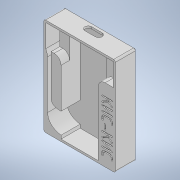
# Autodesk Inventor part: Корпус
Saved by Autodesk Inventor 2021.2 (Build 252289000, 289)
## iProperties
Created: 2023-10-18
Part Number: Корпус
Material: Типовые
Document SubType Name: Modeling
Designer: DELL
Density: 1 g/cm^3
Appearance: По умолчанию
Author: DELL
Autodesk Inventor part; units mm, degrees
ref_plane "YZ Plane" through (0, 0, 0) normal (1, 0, 0) x (0, 1, 0)
ref_plane "XZ Plane" through (0, 0, 0) normal (0, 1, 0) x (-1, 0, 0)
ref_plane "XY Plane" through (0, 0, 0) normal (0, 0, 1) x (1, 0, 0)
sketch "Эскиз1" plane through (0, 0, 0) normal (0, 0, 1) x (1, 0, 0)
  line L0 (10.25, -26.5) -> (-10.25, -26.5) construction
  line L1 (-10.25, -26.5) -> (-10.25, 26.5) construction
  line L2 (-10.25, 26.5) -> (10.25, 26.5) construction
  line L3 (10.25, 26.5) -> (10.25, -26.5) construction
  line L4 (10.25, -26.5) -> (-10.25, 26.5) construction
  line L5 (-10.25, -26.5) -> (10.25, 26.5) construction
  line L6 (19, 14.5) -> (-19, 14.5) construction
  line L7 (-19, 14.5) -> (-19, 26.5) construction
  line L8 (-19, 26.5) -> (19, 26.5) construction
  line L9 (19, 26.5) -> (19, 14.5) construction
  line L10 (19, 14.5) -> (-19, 26.5) construction
  line L11 (-19, 14.5) -> (19, 26.5) construction
  line L12 (-19.5, 14) -> (-14.75, 14)
  arc A0 (-10.75, 10) -> (-14.75, 14) centre (-14.75, 10) ccw
  line L13 (-10.75, 10) -> (-10.75, -27)
  line L14 (-10.75, -27) -> (10.75, -27)
  line L15 (10.75, -27) -> (10.75, 10)
  arc A1 (14.75, 14) -> (10.75, 10) centre (14.75, 10) ccw
  line L16 (14.75, 14) -> (19.5, 14)
  line L17 (19.5, 14) -> (19.5, 27)
  line L18 (19.5, 27) -> (-19.5, 27)
  line L19 (-19.5, 27) -> (-19.5, 14)
  line L20 (0, 26.5) -> (0, -26.5) construction
  line L21 (20.7, -28.2) -> (-20.7, -28.2)
  line L22 (-20.7, -28.2) -> (-20.7, 28.2)
  line L23 (-20.7, 28.2) -> (20.7, 28.2)
  line L24 (20.7, 28.2) -> (20.7, -28.2)
  line L25 (20.7, -28.2) -> (-20.7, 28.2) construction
  line L26 (-20.7, -28.2) -> (20.7, 28.2) construction
  line L27 (-10.75, 10) -> (-10.75, 27)
  line L28 (10.75, 10) -> (10.75, 27)
  point P0 (0, 0)
  point P1 (0, 20.5)
  point P2 (0, 20.5)
  point P3 (0, 0)
  point P4 (0, 0)
  dimension "d0" = 20.5
  dimension "d1" = 53
  dimension "d2" = 38
  dimension "d3" = 12
  dimension "d4" = 0
  dimension "d5" = 0.5
  dimension "d8" = 0.5
  dimension "d9" = 0.5
  dimension "d10" = 0.5
  dimension "d11" = 0.5
  dimension "d12" = 4
  dimension "d13" = 1.2
  dimension "d14" = 1.2
  dimension "d15" = 1.2
  constraints: 58 end point, 11 midpoint, 10 perpendicular, 7 parallel, 5 horizontal, 4 point on circle, 4 tangent, 3 point on line, 2 centre point, 1 vertical alignment, 3 other
  measures "d0" distance of L1.end L2.end
  measures "d1" distance of L0.end L1.end
  measures "d2" distance of L7.end L8.end
  measures "d3" distance of L6.end L7.end
  measures "d4" distance between parallel lines of L2 L8
  measures "d5" distance between parallel lines of L19 L7
  measures "d8" distance between parallel lines of L18 L8
  measures "d9" distance between parallel lines of L6 L12
  measures "d10" distance between parallel lines of L1 L13
  measures "d11" distance between parallel lines of L0 L14
  measures "d12" radius of A0
  measures "d13" distance between parallel lines of L23 L18
  measures "d14" distance between parallel lines of L22 L19
  measures "d15" distance between parallel lines of L14 L21
extrude "Выдавливание1" add sketch "Эскиз1" along normal blind 6 contours L19 L18 L27 A0 L12 | L18 L17 L16 A1 L28 | L21 L22 L23 L24
extrude "Выдавливание2" add sketch "Эскиз1" along normal blind 5 from surface at 6
extrude "Выдавливание3" add sketch "Эскиз1" against normal blind 1 contours L19 L18 L27 A0 L12 | L27 L18 L28 L15 L14 L13 | L18 L17 L16 A1 L28 | L21 L22 L23 L24
fillet "Сопряжение1" radius 1 4 edges at (-20.7, 28.2, 5) (20.7, 28.2, 5) (-20.7, -28.2, 5) (20.7, -28.2, 5)
chamfer "Фаска1" distance 0.5 angle 45 8 edges at (20.7, 0, -1) (20.4071, -27.9071, -1) (0, -28.2, -1) (-20.4071, -27.9071, -1) (-20.7, 0, -1) (-20.4071, 27.9071, -1) (0, 28.2, -1) (20.4071, 27.9071, -1)
sketch "Эскиз2" plane through (-19.7, 28.2, 11) normal (0, 1, 0) x (1, 0, 0)
  line L0 (8.95, 11) -> (30.45, 11) construction
  line L1 (8.95, 11) -> (8.95, 5) construction
  line L2 (30.45, 11) -> (30.45, 5) construction
  line L3 (22.7, 8) -> (16.7, 8) construction
  line L4 (22.7, 10) -> (16.7, 10)
  line L5 (16.7, 6) -> (22.7, 6)
  arc A0 (22.7, 6) -> (22.7, 10) centre (22.7, 8) ccw
  arc A1 (16.7, 10) -> (16.7, 6) centre (16.7, 8) ccw
  point P0 (19.7, 11)
  point P1 (19.7, 8)
  point P2 (19.7, 11)
  dimension "d26" = 10
  dimension "d27" = 4
  dimension "d28" = 1
  constraints: 8 end point, 4 point on circle, 4 tangent, 2 centre point, 2 midpoint, 2 parallel, 1 vertical alignment
  measures "d27" distance between parallel lines of L5 L4
  measures "d28" distance between parallel lines of L4 L0
extrude "Выдавливание4" cut sketch "Эскиз2" against normal up to next
sketch "Эскиз3" plane through (-19.7, 28.2, 11) normal (0, 0, 1) x (1, 0, 0)
  line L0 (38.6265, -20.4965) -> (38.6265, -53.3812) construction
  line L1 (38.6265, -53.3812) -> (33.4814, -53.3812) construction
  line L2 (33.4814, -53.3812) -> (33.4814, -20.4965) construction
  line L3 (33.4814, -20.4965) -> (38.6265, -20.4965) construction
  line L4 (39.4, -56.4) -> (0, -56.4) construction
  line L5 (19.7, -56.4) -> (19.7, 0) construction
  line L6 (16.7, 0) -> (22.7, 0) construction
  line L7 (35.6294, -22.5215) -> (34.8335, -21.8566)
  line L8 (34.8335, -21.8566) -> (32.9093, -21.8566)
  spline S0 degree 2 poles (32.9093, -21.8566) (32.5265, -21.8566) (32.5265, -21.4737) knots 0 0 0 1 1 1
  spline S1 degree 2 poles (32.5265, -21.4737) (32.5265, -21.0909) (32.9093, -21.0909) knots 0 0 0 1 1 1
  line L9 (32.9093, -21.0909) -> (38.2487, -21.0909)
  spline S2 degree 2 poles (38.2487, -21.0909) (38.6265, -21.0909) (38.6265, -21.4737) knots 0 0 0 1 1 1
  spline S3 degree 2 poles (38.6265, -21.4737) (38.6265, -21.8566) (38.2487, -21.8566) knots 0 0 0 1 1 1
  line L10 (38.2487, -21.8566) -> (35.841, -21.8566)
  line L11 (35.841, -21.8566) -> (38.5006, -24.1535)
  spline S4 degree 2 poles (38.5006, -24.1535) (38.6265, -24.2643) (38.6265, -24.4406) knots 0 0 0 1 1 1
  spline S5 degree 2 poles (38.6265, -24.4406) (38.6265, -24.8235) (38.2487, -24.8235) knots 0 0 0 1 1 1
  spline S6 degree 2 poles (38.2487, -24.8235) (38.1027, -24.8235) (37.9616, -24.5968) knots 0 0 0 1 1 1
  line L12 (37.9616, -24.5968) -> (36.1684, -23.0453)
  line L13 (36.1684, -23.0453) -> (33.0957, -24.768)
  spline S7 degree 2 poles (33.0957, -24.768) (33.0051, -24.8235) (32.9093, -24.8235) knots 0 0 0 1 1 1
  spline S8 degree 2 poles (32.9093, -24.8235) (32.7582, -24.8235) (32.5265, -24.5867) (32.5265, -24.4406) knots 0 0 0 1 2 2 2
  spline S9 degree 2 poles (32.5265, -24.4406) (32.5265, -24.2089) (32.7733, -24.088) knots 0 0 0 1 1 1
  line L14 (32.7733, -24.088) -> (35.6294, -22.5215)
  spline S10 degree 2 poles (38.6265, -29.1856) (38.6265, -29.5685) (38.2487, -29.5685) knots 0 0 0 1 1 1
  line L15 (38.2487, -29.5685) -> (32.9093, -29.5685)
  spline S11 degree 2 poles (32.9093, -29.5685) (32.5265, -29.5685) (32.5265, -29.1856) knots 0 0 0 1 1 1
  spline S12 degree 2 poles (32.5265, -29.1856) (32.5265, -28.8028) (32.9093, -28.8028) knots 0 0 0 1 1 1
  line L16 (32.9093, -28.8028) -> (36.7779, -28.8028)
  line L17 (36.7779, -28.8028) -> (33.1814, -26.6066)
  spline S13 degree 2 poles (33.1814, -26.6066) (32.8791, -26.6066) (32.7784, -26.5764) knots 0 0 0 1 1 1
  spline S14 degree 2 poles (32.7784, -26.5764) (32.5265, -26.5109) (32.5265, -26.2238) knots 0 0 0 1 1 1
  spline S15 degree 2 poles (32.5265, -26.2238) (32.5265, -25.841) (32.9093, -25.841) knots 0 0 0 1 1 1
  line L18 (32.9093, -25.841) -> (38.2487, -25.841)
  spline S16 degree 2 poles (38.2487, -25.841) (38.6265, -25.841) (38.6265, -26.2238) knots 0 0 0 1 1 1
  spline S17 degree 2 poles (38.6265, -26.2238) (38.6265, -26.6066) (38.2487, -26.6066) knots 0 0 0 1 1 1
  line L19 (38.2487, -26.6066) -> (34.3802, -26.6066)
  line L20 (34.3802, -26.6066) -> (37.9767, -28.8028)
  spline S18 degree 2 poles (37.9767, -28.8028) (38.279, -28.8028) (38.3747, -28.828) knots 0 0 0 1 1 1
  spline S19 degree 2 poles (38.3747, -28.828) (38.6265, -28.8935) (38.6265, -29.1856) knots 0 0 0 1 1 1
  spline S20 degree 2 poles (38.6265, -33.3463) (38.6265, -33.7292) (38.2487, -33.7292) knots 0 0 0 1 1 1
  spline S21 degree 2 poles (38.2487, -33.7292) (37.8659, -33.7292) (37.8659, -33.3463) knots 0 0 0 1 1 1
  line L21 (37.8659, -33.3463) -> (37.8659, -32.1626)
  spline S22 degree 2 poles (37.8659, -32.1626) (37.8659, -31.6992) (37.468, -31.4675) knots 0 0 0 1 1 1
  spline S23 degree 2 poles (37.468, -31.4675) (37.2816, -31.3566) (37.06, -31.3566) knots 0 0 0 1 1 1
  line L22 (37.06, -31.3566) -> (34.0981, -31.3566)
  spline S24 degree 2 poles (34.0981, -31.3566) (33.7606, -31.3566) (33.2871, -31.8301) (33.2871, -32.1626) knots 0 0 0 1 2 2 2
  line L23 (33.2871, -32.1626) -> (33.2871, -33.3463)
  spline S25 degree 2 poles (33.2871, -33.3463) (33.2871, -33.7292) (32.9093, -33.7292) knots 0 0 0 1 1 1
  spline S26 degree 2 poles (32.9093, -33.7292) (32.5265, -33.7292) (32.5265, -33.3463) knots 0 0 0 1 1 1
  line L24 (32.5265, -33.3463) -> (32.5265, -32.1626)
  spline S27 degree 2 poles (32.5265, -32.1626) (32.5265, -31.5078) (33.4433, -30.591) (34.0981, -30.591) knots 0 0 0 1 2 2 2
  line L25 (34.0981, -30.591) -> (37.065, -30.591)
  spline S28 degree 2 poles (37.065, -30.591) (37.7098, -30.591) (38.6265, -31.5078) (38.6265, -32.1626) knots 0 0 0 1 2 2 2
  line L26 (38.6265, -32.1626) -> (38.6265, -33.3463)
  line L27 (34.0075, -37.502) -> (34.0075, -35.1295)
  spline S29 degree 2 poles (34.0075, -35.1295) (34.0075, -34.7467) (34.3903, -34.7467) knots 0 0 0 1 1 1
  spline S30 degree 2 poles (34.3903, -34.7467) (34.7681, -34.7467) (34.7681, -35.1295) knots 0 0 0 1 1 1
  line L28 (34.7681, -35.1295) -> (34.7681, -37.502)
  spline S31 degree 2 poles (34.7681, -37.502) (34.7681, -37.8848) (34.3903, -37.8848) knots 0 0 0 1 1 1
  spline S32 degree 2 poles (34.3903, -37.8848) (34.0075, -37.8848) (34.0075, -37.502) knots 0 0 0 1 1 1
  line L29 (35.6294, -40.3329) -> (34.8335, -39.668)
  line L30 (34.8335, -39.668) -> (32.9093, -39.668)
  spline S33 degree 2 poles (32.9093, -39.668) (32.5265, -39.668) (32.5265, -39.2851) knots 0 0 0 1 1 1
  spline S34 degree 2 poles (32.5265, -39.2851) (32.5265, -38.9023) (32.9093, -38.9023) knots 0 0 0 1 1 1
  line L31 (32.9093, -38.9023) -> (38.2487, -38.9023)
  spline S35 degree 2 poles (38.2487, -38.9023) (38.6265, -38.9023) (38.6265, -39.2851) knots 0 0 0 1 1 1
  spline S36 degree 2 poles (38.6265, -39.2851) (38.6265, -39.668) (38.2487, -39.668) knots 0 0 0 1 1 1
  line L32 (38.2487, -39.668) -> (35.841, -39.668)
  line L33 (35.841, -39.668) -> (38.5006, -41.9649)
  spline S37 degree 2 poles (38.5006, -41.9649) (38.6265, -42.0757) (38.6265, -42.252) knots 0 0 0 1 1 1
  spline S38 degree 2 poles (38.6265, -42.252) (38.6265, -42.6348) (38.2487, -42.6348) knots 0 0 0 1 1 1
  spline S39 degree 2 poles (38.2487, -42.6348) (38.1027, -42.6348) (37.9616, -42.4082) knots 0 0 0 1 1 1
  line L34 (37.9616, -42.4082) -> (36.1684, -40.8567)
  line L35 (36.1684, -40.8567) -> (33.0957, -42.5794)
  spline S40 degree 2 poles (33.0957, -42.5794) (33.0051, -42.6348) (32.9093, -42.6348) knots 0 0 0 1 1 1
  spline S41 degree 2 poles (32.9093, -42.6348) (32.7582, -42.6348) (32.5265, -42.3981) (32.5265, -42.252) knots 0 0 0 1 2 2 2
  spline S42 degree 2 poles (32.5265, -42.252) (32.5265, -42.0203) (32.7733, -41.8994) knots 0 0 0 1 1 1
  line L36 (32.7733, -41.8994) -> (35.6294, -40.3329)
  spline S43 degree 2 poles (38.6265, -46.997) (38.6265, -47.3799) (38.2487, -47.3799) knots 0 0 0 1 1 1
  line L37 (38.2487, -47.3799) -> (32.9093, -47.3799)
  spline S44 degree 2 poles (32.9093, -47.3799) (32.5265, -47.3799) (32.5265, -46.997) knots 0 0 0 1 1 1
  spline S45 degree 2 poles (32.5265, -46.997) (32.5265, -46.6142) (32.9093, -46.6142) knots 0 0 0 1 1 1
  line L38 (32.9093, -46.6142) -> (36.7779, -46.6142)
  line L39 (36.7779, -46.6142) -> (33.1814, -44.418)
  spline S46 degree 2 poles (33.1814, -44.418) (32.8791, -44.418) (32.7784, -44.3878) knots 0 0 0 1 1 1
  spline S47 degree 2 poles (32.7784, -44.3878) (32.5265, -44.3223) (32.5265, -44.0352) knots 0 0 0 1 1 1
  spline S48 degree 2 poles (32.5265, -44.0352) (32.5265, -43.6524) (32.9093, -43.6524) knots 0 0 0 1 1 1
  line L40 (32.9093, -43.6524) -> (38.2487, -43.6524)
  spline S49 degree 2 poles (38.2487, -43.6524) (38.6265, -43.6524) (38.6265, -44.0352) knots 0 0 0 1 1 1
  spline S50 degree 2 poles (38.6265, -44.0352) (38.6265, -44.418) (38.2487, -44.418) knots 0 0 0 1 1 1
  line L41 (38.2487, -44.418) -> (34.3802, -44.418)
  line L42 (34.3802, -44.418) -> (37.9767, -46.6142)
  spline S51 degree 2 poles (37.9767, -46.6142) (38.279, -46.6142) (38.3747, -46.6394) knots 0 0 0 1 1 1
  spline S52 degree 2 poles (38.3747, -46.6394) (38.6265, -46.7049) (38.6265, -46.997) knots 0 0 0 1 1 1
  spline S53 degree 2 poles (38.6265, -51.1577) (38.6265, -51.5405) (38.2487, -51.5405) knots 0 0 0 1 1 1
  spline S54 degree 2 poles (38.2487, -51.5405) (37.8659, -51.5405) (37.8659, -51.1577) knots 0 0 0 1 1 1
  line L43 (37.8659, -51.1577) -> (37.8659, -49.974)
  spline S55 degree 2 poles (37.8659, -49.974) (37.8659, -49.5106) (37.468, -49.2789) knots 0 0 0 1 1 1
  spline S56 degree 2 poles (37.468, -49.2789) (37.2816, -49.168) (37.06, -49.168) knots 0 0 0 1 1 1
  line L44 (37.06, -49.168) -> (34.0981, -49.168)
  spline S57 degree 2 poles (34.0981, -49.168) (33.7606, -49.168) (33.2871, -49.6415) (33.2871, -49.974) knots 0 0 0 1 2 2 2
  line L45 (33.2871, -49.974) -> (33.2871, -51.1577)
  spline S58 degree 2 poles (33.2871, -51.1577) (33.2871, -51.5405) (32.9093, -51.5405) knots 0 0 0 1 1 1
  spline S59 degree 2 poles (32.9093, -51.5405) (32.5265, -51.5405) (32.5265, -51.1577) knots 0 0 0 1 1 1
  line L46 (32.5265, -51.1577) -> (32.5265, -49.974)
  spline S60 degree 2 poles (32.5265, -49.974) (32.5265, -49.3192) (33.4433, -48.4024) (34.0981, -48.4024) knots 0 0 0 1 2 2 2
  line L47 (34.0981, -48.4024) -> (37.065, -48.4024)
  spline S61 degree 2 poles (37.065, -48.4024) (37.7098, -48.4024) (38.6265, -49.3192) (38.6265, -49.974) knots 0 0 0 1 2 2 2
  line L48 (38.6265, -49.974) -> (38.6265, -51.1577)
  point P0 (19.7, -28.2)
  constraints: 2 end point, 2 midpoint, 2 other
emboss "Рельеф1" sketch "Эскиз3" operation cut depth 0.6 direction (0, 0, -1)
sketch "Эскиз4" plane through (-19.7, 28.2, 11) normal (0, 0, 1) x (1, 0, 0)
  line L0 (8.95, -18.2) -> (8.95, -55.2) construction
  line L1 (0.2, -1.2) -> (0.2, -14.2) construction
  line L2 (0.2, -1.2) -> (3.2, -1.2)
  line L3 (8.95, -1.2) -> (0.2, -1.2) construction
  line L4 (3.2, -1.2) -> (3.2, -14.2)
  line L5 (0.2, -14.2) -> (4.95, -14.2) construction
  line L6 (0.2, -14.2) -> (3.2, -14.2) construction
  line L7 (0.2, -14.2) -> (0.2, -1.2)
  line L8 (8.95, -55.2) -> (30.45, -55.2) construction
  line L9 (1.2, -17.8192) -> (1.2, -45.7113)
  line L10 (3.2, -37.8219) -> (3.2, -14.2)
  line L11 (1.2, -17.8192) -> (1.2, -16.0429) construction
  line L12 (1.2, -16.0429) -> (0.2, -15.3575) construction
  line L13 (0.2, -15.3575) -> (0.2, -14.2) construction
  spline S0 degree 3 poles (1.2, -17.8192) (1.2, -16.0429) (0.2, -15.3575) (0.2, -14.2) knots 1 1 1 1 2 2 2 2
  line L14 (8.95, -53.2) -> (3.0919, -52.2989) construction
  line L15 (3.0919, -52.2989) -> (1.2, -48.7736) construction
  line L16 (1.2, -48.7736) -> (1.2, -45.7113) construction
  spline S1 degree 3 poles (8.95, -53.2) (3.0919, -52.2989) (1.2, -48.7736) (1.2, -45.7113) knots 1 1 1 1 2 2 2 2
  line L17 (8.95, -41.2) -> (4.9393, -41.2) construction
  line L18 (4.9393, -41.2) -> (3.2, -39.7886) construction
  line L19 (3.2, -39.7886) -> (3.2, -37.8219) construction
  spline S2 degree 3 poles (8.95, -41.2) (4.9393, -41.2) (3.2, -39.7886) (3.2, -37.8219) knots 1 1 1 1 2 2 2 2
  line L20 (8.95, -53.2) -> (8.95, -41.2)
  point P0 (19.7, -28.2)
  dimension "d34" = 3
  dimension "d37" = 2
  dimension "d38" = 12
  dimension "d39" = 2
  constraints: 14 end point, 5 point on line, 5 vertical, 3 perpendicular, 1 collinear, 1 horizontal, 9 other
  measures "d34" distance of L1.start L2.end
  measures "d37" distance from line of L14.start L8
  measures "d38" distance of L17.start L14.start
  measures "d39" distance between parallel lines of L9 L10
extrude "Выдавливание5" cut sketch "Эскиз4" against normal up to surface (11 mm away)
equation "\"d8\" = d5"
equation "\"d9\" = d5"
equation "\"d10\" = d5"
equation "\"d11\" = d5"
equation "\"d14\" = d13"
equation "\"d15\" = d13"
